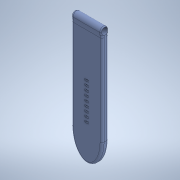
# Autodesk Inventor part: Watch bottom strap
Saved by Autodesk Inventor 2020 (Build 240168000, 168)
## iProperties
Created: 2020-05-08
Part Number: Watch bottom strap
Material: Rubber
Document SubType Name: Modeling
Designer: harry
Density: 0.93 g/cm^3
Appearance: Rubber - Blue
Author: harry
Autodesk Inventor part; units mm, degrees
ref_plane "YZ Plane" through (0, 0, 0) normal (1, 0, 0) x (0, 1, 0)
ref_plane "XZ Plane" through (0, 0, 0) normal (0, 1, 0) x (-1, 0, 0)
ref_plane "XY Plane" through (0, 0, 0) normal (0, 0, 1) x (1, 0, 0)
sketch "Sketch3" plane through (0, 0, 0) normal (1, 0, 0) x (0, 1, 0)
  circle A0 centre (0, 0) radius 3.5
  dimension "d6" = 7
  constraints: 1 centre point, 1 coincident
  measures "d6" diameter of A0
extrude "Extrusion2" add sketch "Sketch3" along normal mid plane 30.5
sketch "Sketch4" plane through (0, 0, 0) normal (1, 0, 0) x (0, 1, 0)
  line L0 (-95, 3.25) -> (-5, 3.25)
  line L1 (-5, 3.25) -> (-5, -3.25)
  line L2 (-5, -3.25) -> (-95, -3.25)
  line L3 (-95, -3.25) -> (-95, 3.25)
  line L4 (-95, 3.25) -> (-5, -3.25) construction
  line L5 (-5, 3.25) -> (-95, -3.25) construction
  circle A0 centre (0, 0) radius 3.5
  arc A1 (-5, 3.25) -> (-0.349127, 3.482544) centre (-5, 49.875) ccw
  arc A2 (-0.349127, -3.482544) -> (-5, -3.25) centre (-5, -49.875) ccw
  point P0 (-50, 0)
  point P1 (-50, 0)
  dimension "d9" = 6.5
  dimension "d12" = 95
  dimension "d13" = 5
  constraints: 12 end point, 6 point on circle, 4 tangent, 3 midpoint, 2 centre point, 2 parallel, 1 horizontal, 1 horizontal alignment, 1 perpendicular
  measures "d9" distance between parallel lines of L2 L0
  measures "d12" distance from line of point (0, 0) L3
  measures "d13" distance from line of L1 point (0, 0)
extrude "Extrusion3" add sketch "Sketch4" along normal mid plane 30.5 contours L0 L1 L2 L3 | A1 A0 A2 L1
sketch "Sketch6" plane through (0, 0, 0) normal (0, 0, 1) x (1, 0, 0)
  line L0 (-15.25, -95) -> (15.25, -95) projected
  ellipse E0 centre (0, -95) end of major axis (0, -120) minor radius 15.25
  point P0 (0, 0)
  dimension "d19" = 25
  constraints: 1 midpoint, 3 other
extrude "Extrusion5" add sketch "Sketch6" along normal mid plane 6.5 contours L0 E0 picked at (-4.951319, -99.580203)
sketch "Sketch7" plane through (-15.25, -5, 3.25) normal (0, 0, 1) x (1, 0, 0)
  line L0 (13.5, -42.349127) -> (17, -42.349127)
  line L1 (17, -42.349127) -> (17, -44.099127)
  line L2 (17, -44.099127) -> (13.5, -44.099127)
  line L3 (13.5, -44.099127) -> (13.5, -42.349127)
  line L4 (13.5, -42.349127) -> (17, -44.099127) construction
  line L5 (17, -42.349127) -> (13.5, -44.099127) construction
  line L6 (0, 4.650873) -> (30.5, 4.650873)
  line L7 (13.5, -46.849127) -> (17, -46.849127)
  line L8 (17, -46.849127) -> (17, -48.599127)
  line L9 (17, -48.599127) -> (13.5, -48.599127)
  line L10 (13.5, -48.599127) -> (13.5, -46.849127)
  line L11 (13.5, -46.849127) -> (17, -48.599127) construction
  line L12 (17, -46.849127) -> (13.5, -48.599127) construction
  line L13 (13.5, -51.349127) -> (17, -51.349127)
  line L14 (17, -51.349127) -> (17, -53.099127)
  line L15 (17, -53.099127) -> (13.5, -53.099127)
  line L16 (13.5, -53.099127) -> (13.5, -51.349127)
  line L17 (13.5, -51.349127) -> (17, -53.099127) construction
  line L18 (17, -51.349127) -> (13.5, -53.099127) construction
  line L19 (13.5, -55.849127) -> (17, -55.849127)
  line L20 (17, -55.849127) -> (17, -57.599127)
  line L21 (17, -57.599127) -> (13.5, -57.599127)
  line L22 (13.5, -57.599127) -> (13.5, -55.849127)
  line L23 (13.5, -55.849127) -> (17, -57.599127) construction
  line L24 (17, -55.849127) -> (13.5, -57.599127) construction
  line L25 (13.5, -60.349127) -> (17, -60.349127)
  line L26 (17, -60.349127) -> (17, -62.099127)
  line L27 (17, -62.099127) -> (13.5, -62.099127)
  line L28 (13.5, -62.099127) -> (13.5, -60.349127)
  line L29 (13.5, -60.349127) -> (17, -62.099127) construction
  line L30 (17, -60.349127) -> (13.5, -62.099127) construction
  line L31 (13.5, -64.849127) -> (17, -64.849127)
  line L32 (17, -64.849127) -> (17, -66.599127)
  line L33 (17, -66.599127) -> (13.5, -66.599127)
  line L34 (13.5, -66.599127) -> (13.5, -64.849127)
  line L35 (13.5, -64.849127) -> (17, -66.599127) construction
  line L36 (17, -64.849127) -> (13.5, -66.599127) construction
  line L37 (13.5, -69.349127) -> (17, -69.349127)
  line L38 (17, -69.349127) -> (17, -71.099127)
  line L39 (17, -71.099127) -> (13.5, -71.099127)
  line L40 (13.5, -71.099127) -> (13.5, -69.349127)
  line L41 (13.5, -69.349127) -> (17, -71.099127) construction
  line L42 (17, -69.349127) -> (13.5, -71.099127) construction
  line L43 (13.5, -73.849127) -> (17, -73.849127)
  line L44 (17, -73.849127) -> (17, -75.599127)
  line L45 (17, -75.599127) -> (13.5, -75.599127)
  line L46 (13.5, -75.599127) -> (13.5, -73.849127)
  line L47 (13.5, -73.849127) -> (17, -75.599127) construction
  line L48 (17, -73.849127) -> (13.5, -75.599127) construction
  line L49 (13.5, -78.349127) -> (17, -78.349127)
  line L50 (17, -78.349127) -> (17, -80.099127)
  line L51 (17, -80.099127) -> (13.5, -80.099127)
  line L52 (13.5, -80.099127) -> (13.5, -78.349127)
  line L53 (13.5, -78.349127) -> (17, -80.099127) construction
  line L54 (17, -78.349127) -> (13.5, -80.099127) construction
  point P0 (15.25, 5)
  point P1 (15.25, -43.224127)
  point P2 (15.25, -43.224127)
  point P3 (15.25, 4.650873)
  point P4 (15.25, -47.724127)
  point P5 (15.25, -47.724127)
  point P6 (15.25, -52.224127)
  point P7 (15.25, -52.224127)
  point P8 (15.25, -56.724127)
  point P9 (15.25, -56.724127)
  point P10 (15.25, -61.224127)
  point P11 (15.25, -61.224127)
  point P12 (15.25, -65.724127)
  point P13 (15.25, -65.724127)
  point P14 (15.25, -70.224127)
  point P15 (15.25, -70.224127)
  point P16 (15.25, -74.724127)
  point P17 (15.25, -74.724127)
  point P18 (15.25, -79.224127)
  point P19 (15.25, -79.224127)
  dimension "d22" = 3.5
  dimension "d23" = 1.75
  dimension "d24" = 47
  dimension "d27" = 4.5
  constraints: 108 end point, 20 midpoint, 2 parallel, 1 collinear, 1 horizontal, 1 perpendicular, 1 vertical, 1 vertical alignment, 95 other
  measures "d22" distance of L0.start L0.end
  measures "d23" distance of L2.end L0.start
  measures "d24" distance from line of point (15.25, 4.651) L0
  measures "d27" distance of L0.start L7.start
extrude "Extrusion6" cut sketch "Sketch7" against normal through all
sketch "Sketch8" plane through (15.25, 0, 0) normal (1, 0, 0) x (0, 0, -1)
  arc A0 (3.482544, -0.349127) -> (-3.482544, -0.349127) centre (0, 0) ccw
  constraints: 1 coincident
hole "Hole1" at (15.25, 0, 0) direction (-1, 0, 0) diameter 6.1 end through all
fillet "Fillet2" radius 2 12 edges at (0, -120, 3.25) (-15.25, -50, 3.25) (-15.25, -2.6717, 3.3082) (-15.25, 3.5, 0) (-15.25, -2.6717, -3.3082) (-15.25, -50, -3.25) (0, -120, -3.25) (15.25, -50, -3.25) (15.25, -2.6717, -3.3082) (15.25, 3.5, 0) (15.25, -2.6717, 3.3082) (15.25, -50, 3.25)
body "Solid2"
